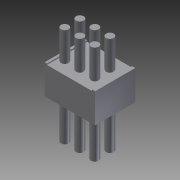
# Autodesk Inventor part: pin_header
Saved by Autodesk Inventor 2012 (Build 160160000, 160)
## iProperties
Created: 2014-09-03
Part Number: pin_header
Material: Default
Document SubType Name: Modeling
Designer: hannes.maierflaig
Density: 1 g/cm^3
Author: hannes.maierflaig
Autodesk Inventor part; units mm, degrees
ref_plane "YZ Plane" through (0, 0, 0) normal (1, 0, 0) x (0, 1, 0)
ref_plane "XZ Plane" through (0, 0, 0) normal (0, 1, 0) x (-1, 0, 0)
ref_plane "XY Plane" through (0, 0, 0) normal (0, 0, 1) x (1, 0, 0)
sketch "Skizze1" plane through (0, 0, 0) normal (0, 0, 1) x (1, 0, 0)
  line L0 (0, 0) -> (4.26, 0)
  line L1 (4.26, 0) -> (4.26, 3.4)
  line L2 (4.26, 3.4) -> (0, 3.4)
  line L3 (0, 3.4) -> (0, 0)
  dimension "d0" = 4.26
  dimension "d1" = 3.4
  constraints: 8 end point, 2 parallel, 1 horizontal, 1 perpendicular
  measures "d0" distance of L2.end L1.end
  measures "d1" distance of L1.end L0.end
extrude "Extrusion1" add sketch "Skizze1" along normal blind 2.5
sketch "Skizze2" plane through (0, 0, 2.5) normal (0, 0, 1) x (1, 0, 0)
  circle A0 centre (0.635, 2.335) radius 0.325
  circle A1 centre (0.635, 1.065) radius 0.325
  circle A2 centre (1.905, 2.335) radius 0.325
  circle A3 centre (1.905, 1.065) radius 0.325
  circle A4 centre (3.175, 1.065) radius 0.325
  circle A5 centre (3.175, 2.335) radius 0.325
  dimension "d4" = 0.65
  dimension "d5" = 0.65
  dimension "d6" = 0.65
  dimension "d7" = 0.65
  dimension "d8" = 0.65
  dimension "d9" = 0.65
  constraints: 9 coincident, 6 centre point
  measures "d4" diameter of A0
  measures "d5" diameter of A1
  measures "d6" diameter of A2
  measures "d7" diameter of A3
  measures "d8" diameter of A4
  measures "d9" diameter of A5
extrude "Extrusion2" add sketch "Skizze2" along normal blind 2.35 and the other way blind 6 separate body
sketch "Skizze3" plane through (0, 3.4, 0) normal (0, 1, 0) x (1, 0, 0)
  line L0 (3.9915, -2.7423) -> (0.1916, -2.7423)
  line L1 (0.1916, -2.7423) -> (0.1916, -2.3884)
  line L2 (0.1916, -2.3884) -> (3.9915, -2.3884)
  line L3 (3.9915, -2.3884) -> (3.9915, -2.7423)
  constraints: 8 end point, 2 parallel, 1 horizontal, 1 perpendicular
extrude "Extrusion3" add sketch "Skizze3" against normal blind 5.15 separate body
combine bodies "Kombinieren1" operation type subtract main body 1 bodies to subtract 3
